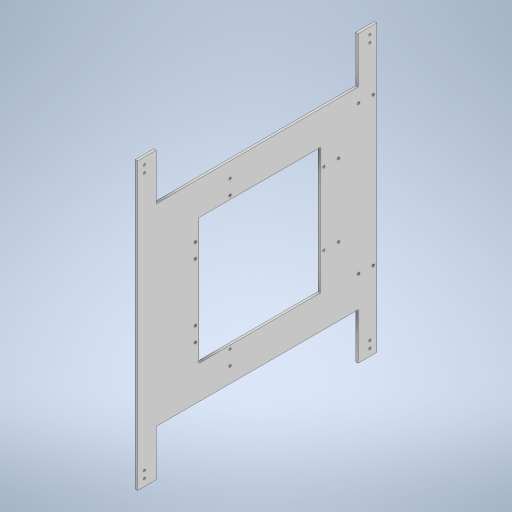
# Autodesk Inventor part: mounting-plate
Saved by Autodesk Inventor 2024 (Build 280153000, 153)
## iProperties
Created: 2023-10-02
Part Number: mounting-plate
Material: Generic
Document SubType Name: Modeling
Designer: Alexander Pollak
Density: 1 g/cm^3
Appearance: Default
Author: Alexander Pollak
Autodesk Inventor part; units mm, degrees
ref_plane "YZ Plane" through (0, 0, 0) normal (1, 0, 0) x (0, 1, 0)
ref_plane "XZ Plane" through (0, 0, 0) normal (0, 1, 0) x (-1, 0, 0)
ref_plane "XY Plane" through (0, 0, 0) normal (0, 0, 1) x (1, 0, 0)
sketch "Sketch2" plane through (0, 0, 0) normal (1, 0, 0) x (0, 1, 0)
  line L0 (-123.45, 103.45) -> (123.45, 103.45)
  line L1 (123.45, 103.45) -> (123.45, -103.45)
  line L2 (123.45, -103.45) -> (-123.45, -103.45)
  line L3 (-123.45, -103.45) -> (-123.45, 103.45)
  line L4 (-123.45, 103.45) -> (123.45, -103.45) construction
  line L5 (123.45, 103.45) -> (-123.45, -103.45) construction
  point P0 (0, 0)
  dimension "d4" = 246.9
  dimension "d5" = 206.9
  constraints: 12 end point, 2 midpoint, 2 parallel, 1 horizontal, 1 perpendicular
  measures "d4" distance of L1.end L2.end
  measures "d5" distance of L0.end L1.end
extrude "Extrusion2" add sketch "Sketch2" along normal blind 2
sketch "Sketch3" plane through (2, 0, 0) normal (1, 0, 0) x (0, 0, -1)
  line L0 (103.45, 123.45) -> (-103.45, 123.45) construction
  line L1 (-103.45, -123.45) -> (103.45, -123.45) construction
  line L2 (-103.45, 123.45) -> (-103.45, -123.45) construction
  line L3 (-53.45, 37.6) -> (-53.45, -37.6) construction
  line L4 (-23.45, -123.45) -> (-23.45, 123.45) construction
  point P0 (0, 0)
  point P1 (-23.45, 70.2)
  point P2 (-23.45, 57.6)
  point P3 (-53.45, 25)
  point P4 (-53.45, -25)
  point P5 (-23.45, -57.6)
  point P6 (-23.45, -70.2)
  dimension "d8" = 12.6
  dimension "d9" = 12.6
  dimension "d10" = 12.6
  dimension "d11" = 12.6
  dimension "d15" = 53.25
  dimension "d24" = 50
  dimension "d25" = 80
  dimension "d26" = 0
  dimension "d27" = 0
  dimension "d28" = 20
  dimension "d29" = 50
  dimension "d30" = 20
  constraints: 4 end point, 2 point on line, 1 perpendicular, 1 vertical
  measures "d8" distance of point (-23.45, 57.6) point (-23.45, 70.2)
  measures "d9" distance of point (-53.45, 25) L3.start
  measures "d10" distance of L3.end point (-53.45, -25)
  measures "d11" distance of point (-23.45, -70.2) point (-23.45, -57.6)
  measures "d15" distance from line of L1 point (-23.45, -70.2)
  measures "d24" distance between parallel lines of L3 L2
  measures "d25" distance between parallel lines of L4 L2
  measures "d26" distance from line of L4 point (-23.45, -70.2)
  measures "d27" distance from line of L4 point (-23.45, 57.6)
  measures "d28" vertical distance of L3.end point (-23.45, -57.6)
  measures "d29" distance of point (-53.45, 25) point (-53.45, -25)
  measures "d30" vertical distance of point (-23.45, 57.6) L3.start
hole "mounting of front power splitters" at (2, 70.2, 23.45) at (2, 57.6, 23.45) at (2, 37.6, 53.45) at (2, 25, 53.45) at (2, -25, 53.45) at (2, -37.6, 53.45) at (2, -57.6, 23.45) at (2, -70.2, 23.45) direction (-1, 0, 0) diameter 2.013 end through all thread size "M2.5x0.45" class "6H" standard "ISO Metric profile"
sketch "Sketch4" plane through (2, 0, 0) normal (1, 0, 0) x (0, 0, -1)
  line L0 (-103.45, 123.45) -> (-103.45, -123.45) construction
  line L1 (-103.45, -56.75) -> (103.45, -56.75) construction
  line L2 (103.45, -123.45) -> (103.45, 123.45) construction
  line L3 (-103.45, -24.15) -> (103.45, -24.15) construction
  line L4 (-103.45, 38.45) -> (103.45, 38.45) construction
  line L5 (-103.45, 71.05) -> (103.45, 71.05) construction
  line L6 (-103.45, -123.45) -> (103.45, -123.45) construction
  point P0 (0, 0)
  point P1 (100.35, -56.75)
  point P2 (87.75, -56.75)
  point P3 (70.35, -24.15)
  point P4 (57.75, -24.15)
  point P5 (70.35, 38.45)
  point P6 (57.75, 38.45)
  point P7 (100.35, 71.05)
  point P8 (87.75, 71.05)
  dimension "d32" = 66.7
  dimension "d33" = 32.6
  dimension "d34" = 62.6
  dimension "d35" = 32.6
  dimension "d36" = 12.6
  dimension "d37" = 12.6
  dimension "d38" = 12.6
  dimension "d39" = 12.6
  dimension "d40" = 3.1
  dimension "d41" = 33.1
  dimension "d42" = 33.1
  dimension "d43" = 3.1
  constraints: 14 point on line, 8 end point, 2 horizontal, 2 perpendicular
  measures "d32" distance between parallel lines of L1 L6
  measures "d33" distance between parallel lines of L1 L3
  measures "d34" distance between parallel lines of L4 L3
  measures "d35" distance between parallel lines of L4 L5
  measures "d36" distance of point (100.35, 71.05) point (87.75, 71.05)
  measures "d37" distance of point (70.35, 38.45) point (57.75, 38.45)
  measures "d38" distance of point (70.35, -24.15) point (57.75, -24.15)
  measures "d39" distance of point (100.35, -56.75) point (87.75, -56.75)
  measures "d40" distance of L1.end point (100.35, -56.75)
  measures "d41" distance from line of L2 point (70.35, -24.15)
  measures "d42" distance from line of L2 point (70.35, 38.45)
  measures "d43" distance from line of L2 point (100.35, 71.05)
hole "mounting of rear power splitters" at (2, -56.75, -100.35) at (2, -56.75, -87.75) at (2, -24.15, -70.35) at (2, -24.15, -57.75) at (2, 38.45, -70.35) at (2, 38.45, -57.75) at (2, 71.05, -100.35) at (2, 71.05, -87.75) direction (-1, 0, 0) diameter 2.013 end through all thread size "M2.5x0.45" class "6H" standard "ISO Metric profile"
sketch "Sketch5" plane through (2, 0, 0) normal (1, 0, 0) x (0, 0, -1)
  line L0 (-103.45, -123.45) -> (103.45, -123.45) projected
  line L1 (-87.25, -83.45) -> (87.25, -83.45)
  line L2 (87.25, -83.45) -> (87.25, -123.45)
  line L3 (87.25, -123.45) -> (-87.25, -123.45)
  line L4 (-87.25, -123.45) -> (-87.25, -83.45)
  line L5 (-87.25, -83.45) -> (87.25, -123.45) construction
  line L6 (87.25, -83.45) -> (-87.25, -123.45) construction
  line L7 (-103.45, 123.45) -> (-103.45, -123.45) projected
  line L8 (103.45, -123.45) -> (103.45, 123.45) projected
  line L9 (-87.25, 83.45) -> (87.25, 83.45)
  line L10 (87.25, 83.45) -> (87.25, 123.45)
  line L11 (87.25, 123.45) -> (-87.25, 123.45)
  line L12 (-87.25, 123.45) -> (-87.25, 83.45)
  line L13 (-87.25, 83.45) -> (87.25, 123.45) construction
  line L14 (87.25, 83.45) -> (-87.25, 123.45) construction
  line L15 (103.45, 123.45) -> (-103.45, 123.45) projected
  point P0 (0, 0)
  point P1 (0, -103.45)
  point P2 (0, 103.45)
  point P3 (87.25, 103.45)
  dimension "d51" = 16.2
  dimension "d52" = 16.2
  dimension "d53" = 40
  dimension "d54" = 16.2
  dimension "d55" = 16.2
  dimension "d56" = 40
  dimension "d57" = 0
  constraints: 24 end point, 5 midpoint, 4 parallel, 2 horizontal, 2 perpendicular, 1 point on line
  measures "d51" distance between parallel lines of L7 L4
  measures "d52" distance between parallel lines of L8 L2
  measures "d53" distance between parallel lines of L0 L1
  measures "d54" distance between parallel lines of L7 L12
  measures "d55" distance from line of L8 point (87.25, 103.45)
  measures "d56" distance between parallel lines of L15 L9
  measures "d57" distance between parallel lines of L15 L11
extrude "Extrusion3" cut sketch "Sketch5" against normal blind 2 contours L4 L1 L2 L0 | L11 L10 L9 L12
sketch "Sketch6" plane through (2, 0, 0) normal (1, 0, 0) x (0, 0, -1)
  line L0 (-50.35, 54.5) -> (54.65, 54.5)
  line L1 (54.65, 54.5) -> (54.65, -54.5)
  line L2 (54.65, -54.5) -> (-50.35, -54.5)
  line L3 (-50.35, -54.5) -> (-50.35, 54.5)
  line L4 (103.45, -123.45) -> (103.45, 123.45) projected
  line L5 (103.45, 123.45) -> (87.25, 123.45) projected
  point P0 (0, 0)
  dimension "d60" = 105
  dimension "d61" = 109
  dimension "d62" = 48.8
  dimension "d63" = 68.95
  constraints: 8 end point, 2 parallel, 1 horizontal, 1 perpendicular
  measures "d60" distance of L1.end L2.end
  measures "d61" distance of L0.end L1.end
  measures "d62" distance between parallel lines of L4 L1
  measures "d63" distance between parallel lines of L0 L5
extrude "Extrusion4" cut sketch "Sketch6" against normal blind 2
sketch "Sketch7" plane through (2, 0, 0) normal (1, 0, 0) x (0, 0, -1)
  line L0 (87.25, -123.45) -> (103.45, -123.45) construction
  line L1 (97.5, -123.45) -> (97.5, 123.45) construction
  line L2 (103.45, 123.45) -> (87.25, 123.45) construction
  line L3 (103.45, -123.45) -> (103.45, 123.45) construction
  line L4 (-87.25, 123.45) -> (-103.45, 123.45) construction
  line L5 (-97.5, 123.45) -> (-97.5, -123.45) construction
  line L6 (-103.45, 123.45) -> (-103.45, -123.45) construction
  line L7 (-103.45, -123.45) -> (-87.25, -123.45) construction
  point P0 (0, 0)
  point P1 (-97.5, -117.45)
  point P2 (-97.5, -111.45)
  point P3 (97.5, -117.45)
  point P4 (97.5, -111.45)
  point P5 (-97.5, 117.45)
  point P6 (-97.5, 111.45)
  point P7 (97.5, 117.45)
  point P8 (97.5, 111.45)
  dimension "d66" = 5.95
  dimension "d67" = 5.95
  dimension "d68" = 6
  dimension "d69" = 6
  dimension "d70" = 6
  dimension "d71" = 6
  dimension "d72" = 6
  dimension "d73" = 6
  dimension "d74" = 6
  dimension "d75" = 6
  constraints: 11 point on line, 4 end point, 2 vertical
  measures "d66" distance between parallel lines of L3 L1
  measures "d67" distance between parallel lines of L6 L5
  measures "d68" distance from line of point (-97.5, 117.45) L4
  measures "d69" distance of point (-97.5, 111.45) point (-97.5, 117.45)
  measures "d70" distance from line of point (97.5, 117.45) L2
  measures "d71" distance of point (97.5, 117.45) point (97.5, 111.45)
  measures "d72" distance from line of L0 point (97.5, -117.45)
  measures "d73" distance of point (97.5, -117.45) point (97.5, -111.45)
  measures "d74" distance from line of L7 point (-97.5, -117.45)
  measures "d75" distance of point (-97.5, -111.45) point (-97.5, -117.45)
hole "Hole3" at (2, -117.45, 97.5) at (2, -111.45, 97.5) at (2, -117.45, -97.5) at (2, -111.45, -97.5) at (2, 117.45, 97.5) at (2, 111.45, 97.5) at (2, 117.45, -97.5) at (2, 111.45, -97.5) direction (-1, 0, 0) diameter 2.013 end through all thread size "M2.5x0.45" class "6H" standard "ISO Metric profile"
body "Solid2"
